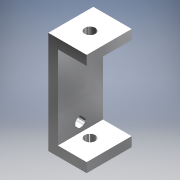
# Autodesk Inventor part: Extrusion ends
Saved by Autodesk Inventor 2019.4 (Build 234330000, 330)
## iProperties
Created: 2020-01-03
Part Number: Extrusion ends
Material: Aluminum 6061
Document SubType Name: Modeling
Designer: Mark
Mass: 16.3314 g
Surface Area: 33.6225 cm^2
Volume: 6.04867 cm^3
Density: 2.7 g/cm^3
Appearance: Aluminum - Flat
Author: Mark
Autodesk Inventor part; units mm, degrees
ref_plane "YZ Plane" through (0, 0, 0) normal (1, 0, 0) x (0, 1, 0)
ref_plane "XZ Plane" through (0, 0, 0) normal (0, 1, 0) x (-1, 0, 0)
ref_plane "XY Plane" through (0, 0, 0) normal (0, 0, 1) x (1, 0, 0)
sketch "Sketch1" plane through (0, 0, 0) normal (1, 0, 0) x (0, 1, 0)
  line L0 (-26.75, 11.75) -> (26.75, 11.75)
  line L1 (26.75, 11.75) -> (26.75, -11.75)
  line L2 (26.75, -11.75) -> (-26.75, -11.75)
  line L3 (-26.75, -11.75) -> (-26.75, 11.75)
  line L4 (-26.75, 11.75) -> (26.75, -11.75) construction
  line L5 (26.75, 11.75) -> (-26.75, -11.75) construction
  circle A0 centre (16.75, 0) radius 2.75
  circle A1 centre (-16.75, 0) radius 2.75
  point P0 (0, 0)
  dimension "d0" = 53.5
  dimension "d1" = 23.5
  dimension "d2" = 5.5
  dimension "d3" = 5.5
  dimension "d4" = 10
  dimension "d5" = 10
  dimension "d6" = 11.75
  dimension "d7" = 11.75
  constraints: 12 end point, 2 centre point, 2 midpoint, 2 parallel, 1 horizontal, 1 perpendicular
  measures "d0" distance of L1.end L2.end
  measures "d1" distance of L0.end L1.end
  measures "d2" diameter of A0
  measures "d3" diameter of A1
  measures "d4" distance from line of L3 A1.centre
  measures "d5" distance from line of L1 A0.centre
  measures "d6" distance from line of L2 A0.centre
  measures "d7" distance from line of L2 A1.centre
extrude "Extrusion1" add sketch "Sketch1" along normal blind 5
sketch "Sketch2" plane through (5, 0, 0) normal (1, 0, 0) x (0, 0, -1)
  line L0 (-11.75, 26.75) -> (-11.75, -26.75) projected
  line L1 (-11.75, 26.75) -> (11.75, 26.75)
  line L2 (11.75, 26.75) -> (11.75, 21.75)
  line L3 (11.75, 21.75) -> (-11.75, 21.75)
  line L4 (-11.75, 21.75) -> (-11.75, 26.75)
  line L5 (-11.75, -26.75) -> (11.75, -26.75) projected
  line L6 (-11.75, -26.75) -> (11.75, -26.75)
  line L7 (11.75, -26.75) -> (11.75, -21.75)
  line L8 (11.75, -21.75) -> (-11.75, -21.75)
  line L9 (-11.75, -21.75) -> (-11.75, -26.75)
  point P0 (0, 0)
  dimension "d10" = 23.5
  dimension "d11" = 5
  dimension "d12" = 23.5
  dimension "d13" = 5
  constraints: 16 end point, 4 parallel, 2 horizontal, 2 perpendicular
  measures "d10" distance of L2.end L3.end
  measures "d11" distance of L1.end L2.end
  measures "d12" distance of L8.end L7.end
  measures "d13" distance of L7.end L6.end
extrude "Extrusion2" add sketch "Sketch2" along normal blind 15
sketch "Sketch3" plane through (0, 26.75, 11.75) normal (0, 1, 0) x (1, 0, 0)
  circle A0 centre (10, 11.75) radius 2.75
  line L0 (0, 0) -> (0, 23.5) projected
  line L1 (0, 0) -> (20, 0) projected
  point P0 (0, 11.75)
  dimension "d16" = 5.5
  dimension "d17" = 10
  dimension "d18" = 11.75
  constraints: 1 centre point
  measures "d16" diameter of A0
  measures "d17" distance from line of L0 A0.centre
  measures "d18" distance from line of L1 A0.centre
extrude "Extrusion3" cut sketch "Sketch3" against normal up to surface (53.5 mm away)
body "Solid1"
